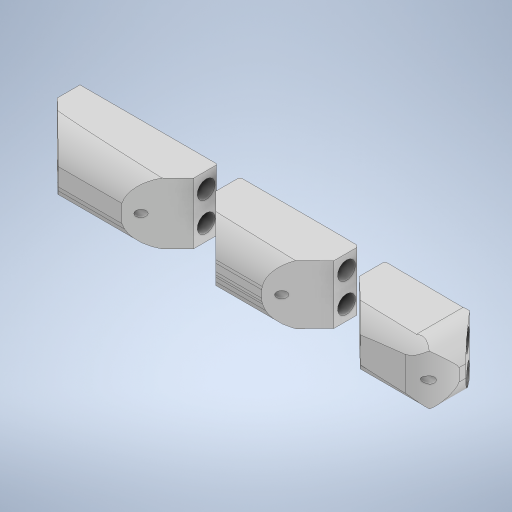
# Autodesk Inventor part: Finger_Ring
Saved by Autodesk Inventor 2024 (Build 280153000, 153)
## iProperties
Created: 2025-05-19
Part Number: Finger_Ring
Material: Generic
Document SubType Name: Modeling
Designer: Mehdi Charfeddine
Density: 1 g/cm^3
Appearance: Default
Author: Mehdi Charfeddine
Autodesk Inventor part; units mm, degrees
ref_plane "YZ Plane" through (0, 0, 0) normal (1, 0, 0) x (0, 1, 0)
ref_plane "XZ Plane" through (0, 0, 0) normal (0, 1, 0) x (-1, 0, 0)
ref_plane "XY Plane" through (0, 0, 0) normal (0, 0, 1) x (1, 0, 0)
sketch "Sketch1" plane through (0, 0, 0) normal (1, 0, 0) x (0, 1, 0)
  line L0 (406.5258, 186.3932) -> (406.5258, 12.8725)
  line L1 (406.5258, 12.8725) -> (393.6246, 0)
  line L2 (393.6246, 0) -> (374.7029, 0)
  line L3 (374.7029, 0) -> (82.6155, 0)
  line L4 (82.6155, 0) -> (63.5884, 0)
  line L5 (63.5884, 0) -> (50.7445, 12.8725)
  line L6 (50.7445, 12.8725) -> (51.2145, 186.9471)
  arc A0 (68.0929, 256.237) -> (51.2145, 186.9471) centre (203.5684, 186.5358) ccw
  arc A1 (110.057, 307.9965) -> (68.0929, 256.237) centre (210.155, 183.9508) ccw
  arc A2 (152.5787, 332.4554) -> (110.057, 307.9965) centre (209.9723, 183.4857) ccw
  arc A3 (183.2788, 340.7945) -> (152.5787, 332.4554) centre (208.0822, 188.8023) ccw
  arc A4 (195.7582, 342.341) -> (183.2788, 340.7945) centre (207.5276, 196.2401) ccw
  arc A5 (212.8849, 342.9077) -> (195.7582, 342.341) centre (220.6385, -150.4622) ccw
  line L7 (212.8849, 342.9077) -> (241.7888, 342.9077)
  line L8 (241.7888, 342.9077) -> (242.0073, 344.8164)
  arc A6 (241.7888, 342.9077) -> (246.3102, 342.9077) centre (244.0495, 724.731) ccw
  arc A7 (268.7679, 341.5543) -> (246.3102, 342.9077) centre (249.0701, 201.7031) ccw
  arc A8 (406.5258, 186.3932) -> (268.7679, 341.5543) centre (247.4402, 183.8849) ccw
  arc A9 (339.7711, 25.3914) -> (346.7092, 108.7449) centre (310.8261, 69.7662) ccw
  circle A10 centre (310.8261, 69.7662) radius 50
  arc A11 (97.5109, 89.9944) -> (115.2466, 26.6397) centre (146.5021, 69.5492) ccw
  circle A12 centre (146.5021, 69.5492) radius 50
  arc A13 (246.3102, 298.3793) -> (210.7895, 298.3793) centre (228.5498, 286.8439) ccw
  circle A14 centre (228.5498, 286.8439) radius 20
  point P0 (0, 0)
  dimension "d0" = 100
  dimension "d1" = 100
  dimension "d2" = 40
  constraints: 24 point on circle, 18 end point, 15 centre point, 3 coincident, 3 point on line, 2 perpendicular, 1 horizontal, 1 tangent, 1 vertical
  measures "d0" diameter of A10
  measures "d1" diameter of A12
  measures "d2" diameter of A14
extrude "Extrusion1" add sketch "Sketch1" along normal mid plane 4000
sketch "Sketch2" plane through (0, 0, 0) normal (0, 0, 1) x (1, 0, 0)
  line L0 (-736.6005, 406.4005) -> (-736.6005, 50.8326)
  line L1 (-736.6005, 50.8326) -> (25.5842, 57.5058)
  line L2 (25.5842, 57.5058) -> (25.5842, 399.4141)
  line L3 (25.5842, 399.4141) -> (-736.6005, 406.4005)
  line L4 (149.4559, 398.2787) -> (810.0593, 392.2234)
  line L5 (810.0593, 392.2234) -> (810.0593, 64.3742)
  line L6 (810.0593, 64.3742) -> (152.4298, 58.6164)
  line L7 (152.4298, 58.6164) -> (149.4559, 398.2787)
  line L8 (955.304, 390.892) -> (952.3225, 65.6197)
  line L9 (952.3225, 65.6197) -> (1388.5629, 69.4392)
  line L10 (1388.5629, 69.4392) -> (1391.4728, 386.894)
  line L11 (1391.4728, 386.894) -> (955.304, 390.892)
  arc A0 (1548.5348, 263.5186) -> (1391.4728, 386.894) centre (1418.7874, 260.0058) ccw
  arc A1 (1388.5629, 69.4392) -> (1548.5348, 193.6021) centre (1418.0274, 196.6126) ccw
  line L12 (1548.5348, 193.6021) -> (1548.5348, 263.5186)
  line L13 (-2215.632, 732.4701) -> (2205.1038, 732.4701)
  line L14 (2205.1038, 732.4701) -> (2205.1038, -729.6854)
  line L15 (2205.1038, -729.6854) -> (-2215.632, -729.6854)
  line L16 (-2215.632, -729.6854) -> (-2215.632, 732.4701)
  point P0 (0, 0)
  constraints: 34 end point, 8 point on line, 5 parallel, 4 point on circle, 3 perpendicular, 2 centre point, 2 vertical, 1 horizontal
extrude "Extrusion2" cut sketch "Sketch2" along normal mid plane 4000
sketch "Sketch3" plane through (0, 0, 0) normal (0, 1, 0) x (-1, 0, 0)
  line L0 (724.1444, 0) -> (-12.178, 0)
  line L1 (-12.178, 0) -> (-25.7075, 12.4264)
  line L2 (-25.7075, 12.4264) -> (-25.7075, 139.9906)
  line L3 (-25.7075, 139.9906) -> (175.0513, 340.1491)
  line L4 (175.0513, 340.1491) -> (530.742, 340.1491)
  line L5 (530.742, 340.1491) -> (736.6092, 139.7319)
  line L6 (736.6092, 139.7319) -> (736.6092, 12.8037)
  line L7 (736.6092, 12.8037) -> (724.1444, 0)
  line L8 (-162.4377, 0) -> (-149.6293, 13.9454)
  line L9 (-149.6293, 13.9454) -> (-149.6293, 139.7319)
  line L10 (-149.6293, 139.7319) -> (-352.1774, 342.8875)
  line L11 (-352.1774, 342.8875) -> (-609.6432, 342.8875)
  line L12 (-609.6432, 342.8875) -> (-810.2946, 139.7319)
  line L13 (-810.2946, 139.7319) -> (-810.2946, 12.8037)
  line L14 (-810.2946, 12.8037) -> (-797.331, 0)
  line L15 (-797.331, 0) -> (-162.4377, 0)
  line L16 (-952.2881, 12.8037) -> (-964.934, 0)
  line L17 (-964.934, 0) -> (-1428.3836, 0)
  line L18 (-1428.3836, 0) -> (-1550.5585, 144.4579)
  line L19 (-1550.5585, 144.4579) -> (-1549.5628, 162.4108)
  arc A0 (-1392.4575, 324.2753) -> (-1549.5628, 162.4108) centre (-1385.9832, 160.8162) ccw
  line L20 (-1392.4575, 324.2753) -> (-1154.8948, 333.6847)
  line L21 (-1154.8948, 333.6847) -> (-952.2881, 139.7319)
  line L22 (-952.2881, 139.7319) -> (-952.2881, 12.8037)
  line L23 (1194.7513, 556.9374) -> (-2078.0894, 556.9374)
  line L24 (-2078.0894, 556.9374) -> (-2078.0894, -491.6053)
  line L25 (-2078.0894, -491.6053) -> (1194.7513, -491.6053)
  line L26 (1194.7513, -491.6053) -> (1194.7513, 556.9374)
  point P0 (0, 0)
  constraints: 54 end point, 8 perpendicular, 4 parallel, 2 horizontal, 2 point on circle, 2 point on line, 2 vertical, 1 centre point
extrude "Extrusion3" cut sketch "Sketch3" along normal mid plane 4000
body "Solid1"
